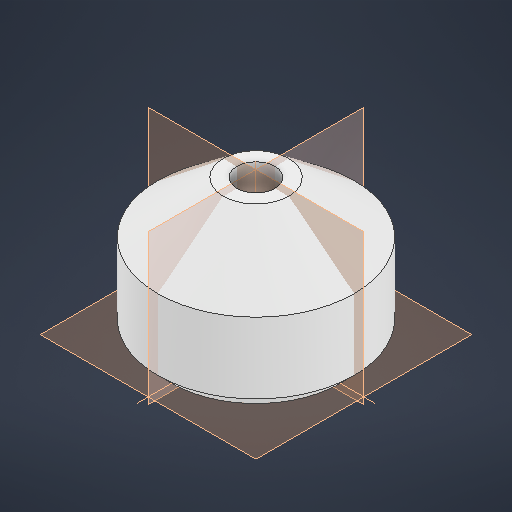
# Autodesk Inventor part: magnet-holder
Saved by Autodesk Inventor 2026.1 (Build 301233020, 233B)
## iProperties
Created: 2024-12-19
Part Number: magnet-holder
Material: PET Plastic
Document SubType Name: Modeling
Designer: yehorderehus
Density: 1.541 g/cm^3
Appearance: Smooth - White
Mass: 0.910312 g
Surface Area: 8.73669 cm^2
Volume: 0.827556 cm^3
Author: yehorderehus
Autodesk Inventor part; units mm, degrees
sketch "Sketch1" plane through (0, 0, 0) normal (0, 0, 1) x (1, 0, 0)
  line L0 (-5.2, 0) -> (-5.2, 5.2)
  line L1 (0, 14.64) -> (0, -2.44) projected
  line L2 (-5.2, 0) -> (-6.2, 0)
  line L3 (-6.2, 0) -> (-7.2, 1)
  line L4 (-8.64, 0) -> (1.44, 0) projected
  line L5 (-7.2, 1) -> (-7.2, 6.2)
  line L6 (-5.2, 5.2) -> (-3.2, 5.2)
  line L7 (-3.2, 5.2) -> (-3.2, 7.6)
  line L8 (-3.2, 7.6) -> (-1.4, 7.6)
  line L9 (0, 7.2) -> (0, 12.2)
  line L10 (-1.4, 10) -> (-2.4, 10)
  line L11 (-2.4, 10) -> (-7.2, 6.2)
  line L12 (0, -2.44) -> (0, 14.64) projected
  line L13 (-1.4, 7.6) -> (-1.4, 10)
  point P0 (0, 0)
  dimension "d0" = 5.2
  dimension "d1" = 5.2
  dimension "d2" = 1
  dimension "d3" = 1
  dimension "d5" = 5.2
  dimension "d6" = 3.2
  dimension "d7" = 2.4
  dimension "d8" = 0
  dimension "d11" = 2.4
  dimension "d21" = 1.4
  dimension "d22" = 2
  dimension "d23" = 2.4
  constraints: 22 end point, 4 horizontal, 4 vertical, 1 perpendicular
  measures "d0" distance between parallel lines of L1 L0
  measures "d1" distance of L0.start L0.end
  measures "d2" distance of L0.start L2.end
  measures "d3" distance from line of L4 L3.end
  measures "d5" distance of L3.end L5.end
  measures "d6" distance from line of L1 L6.end
  measures "d7" distance of L6.end L7.end
  measures "d8" distance from line of L1 L9.start
  measures "d11" distance from line of L1 L10.end
  measures "d21" distance between parallel lines of L9 L13
  measures "d22" distance between parallel lines of L5 L0
  measures "d23" distance between parallel lines of L8 L10
revolve "Revolution1" add sketch "Sketch1" angle 360 about axis through (0, -10, 0) along (0, 1, 0)
body "Solid1"
